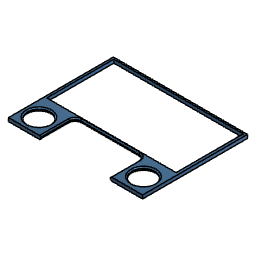
Drive_Through_Testing_Barrier v1 (Autodesk Fusion 360 design; units mm, degrees)
Autodesk Fusion 360 part; units mm, degrees
sketch "Sketch1" plane through (0, 0, 0) normal (0, 1, 0) x (1, 0, 0)
  line L0 (-25, 25) -> (-25, 482)
  line L1 (-25, 482) -> (-609, 482)
  line L2 (-609, 482) -> (-609, 25)
  line L3 (-609, 25) -> (-469, 25)
  line L4 (-444, 175) -> (-190, 175)
  line L5 (-469, 25) -> (-469, 150)
  arc A0 (-444, 175) -> (-469, 150) centre (-444, 150) ccw
  line L6 (-165, 25) -> (-25, 25)
  line L7 (-165, 150) -> (-165, 25)
  arc A1 (-165, 150) -> (-190, 175) centre (-190, 150) ccw
  point P0 (-469, 175)
  point P1 (-165, 175)
  dimension "d1" = 457
  dimension "d2" = 584
  dimension "d3" = 457
  dimension "d5" = 304
  dimension "d7" = 25
  dimension "d8" = 25
  constraint vertical L0
  constraint perpendicular L0 L1
  constraint perpendicular L1 L2
  constraint perpendicular L2 L3
  constraint perpendicular L4 L5
  constraint coincident P0 L4
  constraint coincident P0 L5
  constraint tangent L4 A0
  constraint tangent L5 A0
  constraint perpendicular L0 L6
  constraint perpendicular L6 L7
  constraint coincident P1 L4
  constraint coincident P1 L7
  constraint tangent L4 A1
  constraint tangent L7 A1
  measures "d1" distance of L0.start L0.end
  measures "d2" distance of L0.end L1.end
  measures "d3" distance of L1.end L2.end
  measures "d5" distance of P0 P1
  measures "d7" radius of A0
  measures "d8" radius of A1
extrude "Extrude1" add sketch "Sketch1" along normal blind 15
sketch "Sketch2" plane through (0, 15, 0) normal (0, 1, 0) x (-1, 0, 0)
  line L0 (165, -25) -> (25, -25)
  line L1 (25, -25) -> (25, -482)
  line L2 (25, -482) -> (609, -482)
  line L3 (609, -482) -> (609, -25)
  line L4 (609, -25) -> (469, -25)
  line L5 (469, -25) -> (469, -150)
  arc A0 (444, -175) -> (469, -150) centre (444, -150) ccw
  line L6 (444, -175) -> (190, -175)
  arc A1 (165, -150) -> (190, -175) centre (190, -150) ccw
  line L7 (165, -150) -> (165, -25)
  line L8 (600, -475) -> (36.4384, -475)
  line L9 (36.4384, -475) -> (36.4384, -182.5461)
  line L10 (36.4384, -182.5461) -> (600, -182.5461)
  line L11 (600, -182.5461) -> (600, -475)
  dimension "d11" = 563.5616
  constraint horizontal L8
  constraint vertical L9
  constraint horizontal L10
  constraint vertical L11
  measures "d11" distance of L8.start L8.end
extrude "Extrude2" cut sketch "Sketch2" against normal blind 10 contours L8 L9 L10 L11
shell "Shell1" thickness 5 removed faces 1 at (-412.1461, 5, -377.5154)
extrude "Extrude3" cut 1 faces at (-412.1461, 5, -377.5154) along direction (0, -1, 0) blind 5
sketch "Sketch3" plane through (0, 15, 0) normal (0, 1, 0) x (-1, 0, 0)
  line L0 (36.4384, -475) -> (36.4384, -182.5461)
  line L1 (36.4384, -182.5461) -> (600, -182.5461)
  line L2 (600, -182.5461) -> (600, -475)
  line L3 (600, -475) -> (36.4384, -475)
  line L4 (165, -25) -> (25, -25)
  line L5 (25, -25) -> (25, -482)
  line L6 (25, -482) -> (609, -482)
  line L7 (609, -482) -> (609, -25)
  line L8 (609, -25) -> (469, -25)
  line L9 (469, -25) -> (469, -150)
  arc A0 (444, -175) -> (469, -150) centre (444, -150) ccw
  line L10 (444, -175) -> (190, -175)
  arc A1 (165, -150) -> (190, -175) centre (190, -150) ccw
  line L11 (165, -150) -> (165, -25)
  circle A2 centre (544.2965, -92.6642) radius 50
  circle A3 through (154.0584, -100.5299, -5) (79.0584, -57.2286, -5) (79.0584, -143.8311, -5)
  dimension "d17" = 100
  dimension "d18" = 100
  measures "d17" diameter of A2
extrude "Extrude4" cut sketch "Sketch3" against normal blind 20 contours A2
sketch "Sketch4" plane through (0, 15, 0) normal (0, 1, 0) x (-1, 0, 0)
  circle A0 centre (544.2965, -92.6642) radius 50
  line L0 (36.4384, -475) -> (36.4384, -182.5461)
  line L1 (36.4384, -182.5461) -> (600, -182.5461)
  line L2 (600, -182.5461) -> (600, -475)
  line L3 (600, -475) -> (36.4384, -475)
  line L4 (165, -25) -> (25, -25)
  line L5 (25, -25) -> (25, -482)
  line L6 (25, -482) -> (609, -482)
  line L7 (609, -482) -> (609, -25)
  line L8 (609, -25) -> (469, -25)
  line L9 (469, -25) -> (469, -150)
  arc A1 (444, -175) -> (469, -150) centre (444, -150) ccw
  line L10 (444, -175) -> (190, -175)
  arc A2 (165, -150) -> (190, -175) centre (190, -150) ccw
  line L11 (165, -150) -> (165, -25)
  circle A3 centre (92.6724, -96.5653) radius 50
  dimension "d23" = 100
  measures "d23" diameter of A3
extrude "Extrude5" cut sketch "Sketch4" against normal blind 20 contours A3
fillet "Fillet1" radius 5 1 edges at (-46.056, 0, -114.6461)
fillet "Fillet2" radius 5 1 edges at (-46.056, 15, -78.4846)
fillet "Fillet3" radius 5 1 edges at (-497.6801, 0, -110.745)
fillet "Fillet4" radius 5 1 edges at (-497.6801, 15, -74.5834)
fillet "Fillet5" radius 5 5 edges at (-469, 15, -87.5) (-461.6777, 15, -167.6777) (-317, 15, -175) (-172.3223, 15, -167.6777) (-165, 15, -87.5)
fillet "Fillet6" radius 5 5 edges at (-469, 0, -87.5) (-461.6777, 0, -167.6777) (-317, 0, -175) (-172.3223, 0, -167.6777) (-165, 0, -87.5)
